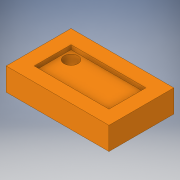
# Autodesk Inventor part: BaseForCanBusConnector
Saved by Autodesk Inventor 2018.1 (Build 221171000, 171)
## iProperties
Created: 2017-10-25
Part Number: BaseForCanBusConnector
Material: Generic
Document SubType Name: Modeling
Designer: steele
Density: 1 g/cm^3
Appearance: Orange
Author: steele
Autodesk Inventor part; units mm, degrees
ref_plane "YZ Plane" through (0, 0, 0) normal (1, 0, 0) x (0, 1, 0)
ref_plane "XZ Plane" through (0, 0, 0) normal (0, 1, 0) x (-1, 0, 0)
ref_plane "XY Plane" through (0, 0, 0) normal (0, 0, 1) x (1, 0, 0)
sketch "Sketch1" plane through (0, 0, 0) normal (0, 1, 0) x (-1, 0, 0)
  line L0 (18.6817, 11.7856) -> (-18.6817, 11.7856)
  line L1 (-18.6817, 11.7856) -> (-18.6817, -11.7856)
  line L2 (-18.6817, -11.7856) -> (18.6817, -11.7856)
  line L3 (18.6817, -11.7856) -> (18.6817, 11.7856)
  line L4 (18.6817, 11.7856) -> (-18.6817, -11.7856) construction
  line L5 (-18.6817, 11.7856) -> (18.6817, -11.7856) construction
  point P0 (0, 0)
  dimension "d0" = 37.3634
  dimension "d1" = 23.5712
  constraints: 12 end point, 2 midpoint, 2 parallel, 1 horizontal, 1 perpendicular
  measures "d0" distance of L1.end L2.end
  measures "d1" distance of L2.end L0.start
extrude "Extrusion1" add sketch "Sketch1" against normal blind 8.255
sketch "Sketch2" plane through (0, 0, 0) normal (0, 1, 0) x (1, 0, 0)
  line L0 (-13.6017, -6.7056) -> (13.6017, -6.7056)
  line L1 (13.6017, -6.7056) -> (13.6017, 6.7056)
  line L2 (13.6017, 6.7056) -> (-13.6017, 6.7056)
  line L3 (-13.6017, 6.7056) -> (-13.6017, -6.7056)
  line L4 (-13.6017, -6.7056) -> (13.6017, 6.7056) construction
  line L5 (13.6017, -6.7056) -> (-13.6017, 6.7056) construction
  point P0 (0, 0)
  dimension "d4" = 13.4112
  dimension "d5" = 27.2034
  constraints: 12 end point, 2 midpoint, 2 parallel, 1 horizontal, 1 perpendicular
  measures "d4" distance of L2.end L0.start
  measures "d5" distance of L1.end L2.end
extrude "Extrusion2" cut sketch "Sketch2" against normal blind 1.6002
sketch "Sketch3" plane through (0, -8.255, 0) normal (0, -1, 0) x (1, 0, 0)
  line L0 (10.4521, 3.556) -> (-10.4521, 3.556) construction
  line L1 (-10.4521, 3.556) -> (-10.4521, -3.556) construction
  line L2 (-10.4521, -3.556) -> (10.4521, -3.556) construction
  line L3 (10.4521, -3.556) -> (10.4521, 3.556) construction
  line L4 (10.4521, 3.556) -> (-10.4521, -3.556) construction
  line L5 (-10.4521, 3.556) -> (10.4521, -3.556) construction
  point P0 (0, 0)
  dimension "d8" = 7.112
  dimension "d9" = 20.9042
  constraints: 12 end point, 4 coincident, 2 midpoint, 2 parallel, 1 horizontal, 1 perpendicular
  measures "d8" distance of L2.end L0.start
  measures "d9" distance of L1.end L2.end
hole "Hole2" at (10.4521, -8.255, -3.556) at (-10.4521, -8.255, -3.556) at (-10.4521, -8.255, 3.556) at (10.4521, -8.255, 3.556) direction (0, 1, 0) diameter 5.08 depth 3.175
sketch "Sketch9" plane through (-10.4521, -5.08, -3.556) normal (0, -1, 0) x (1, 0, 0)
  point P0 (0, 0)
hole "Hole6" at (-10.4521, -5.08, -3.556) direction (0, 1, 0) diameter 5.08 depth 3.4798
equation "\"d0\" = PartWidth"
equation "\"d1\" = PartLength"
equation "\"d2\" = BaseHeight"
equation "\"d4\" = CanBaseLength"
equation "\"d5\" = CanBaseWidth"
equation "\"d8\" = HoleLength"
equation "\"d9\" = HoleWidth"
equation "\"d18\" = boltHeadDiam"
equation "\"d23\" = boltHeadHeight"
equation "\"HoleWidth\" = 20.9042"
equation "\"HoleLength\" = 7.112"
equation "\"BaseOffset\" = 5.08"
equation "\"PartWidth\" = CanBaseWidth + 2 * BaseOffset"
equation "\"PartLength\" = CanBaseLength + 2 * BaseOffset"
equation "\"boardGap\" = 0.508"
equation "\"boltHeadHeight\" = 3.175"
equation "\"boltHeadDiam\" = 5.08"
equation "\"BaseHeight\" = 8.255"
equation "\"CanBaseLength\" = 13.4112"
equation "\"CanBaseWidth\" = 27.2034"
body "Solid1"
